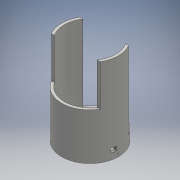
# Autodesk Inventor part: outsideCover
Saved by Autodesk Inventor 2016 (Build 200138000, 138)
## iProperties
Created: 2016-10-27
Part Number: outsideCover
Material: 一般
Document SubType Name: Modeling
Designer: Daisuke
Density: 1 g/cm^3
Appearance: 既定
Author: Daisuke
Autodesk Inventor part; units mm, degrees
ref_plane "XY Plane" through (0, 0, 0) normal (0, 0, 1) x (1, 0, 0)
sketch "スケッチ1" plane through (0, 0, 0) normal (0, 0, 1) x (1, 0, 0)
  circle A0 centre (0, 0) radius 50
  circle A1 centre (0, 0) radius 55
  line L0 (0, 0) -> (47.6314, 27.5) construction
  line L1 (0, 0) -> (55, 0) construction
  line L2 (0, 0) -> (-47.6314, 27.5) construction
  line L3 (0, 0) -> (55, 0) construction
  dimension "d0" = 100
  dimension "d1" = 110
  dimension "d2" = 30
  dimension "d3" = 150
  constraints: 8 end point, 2 centre point, 2 coincident, 2 equal length, 2 horizontal, 2 point on circle
  measures "d0" diameter of A0
  measures "d1" diameter of A1
  measures "d2" angle of L1 L0
  measures "d3" angle of L3 L2
extrude "押し出し1" add sketch "スケッチ1" along normal blind 20
sketch "スケッチ2" plane through (0, 0, 20) normal (0, 0, 1) x (1, 0, 0)
  line L0 (0, 0) -> (47.6314, 27.5) construction
  circle A0 centre (0, 0) radius 55 construction
  line L1 (0, 0) -> (55, 0) construction
  line L2 (0, 0) -> (-47.6314, 27.5) construction
  line L3 (0, 0) -> (55, 0) construction
  line L4 (-47.6314, 27.5) -> (-41.7582, 27.5)
  line L5 (41.7582, 27.5) -> (47.6314, 27.5)
  line L6 (0, 0) -> (47.6314, -27.5) construction
  line L7 (0, 0) -> (55, 0) construction
  line L8 (0, 0) -> (-47.6314, -27.5) construction
  line L9 (0, 0) -> (55, 0) construction
  arc A1 (-47.6314, 27.5) -> (-47.6314, -27.5) centre (0, 0) ccw
  arc A2 (47.6314, -27.5) -> (47.6314, 27.5) centre (0, 0) ccw
  arc A3 (-41.7582, 27.5) -> (-41.7582, -27.5) centre (0, 0) ccw
  arc A4 (41.7582, -27.5) -> (41.7582, 27.5) centre (0, 0) ccw
  line L10 (-47.6314, -27.5) -> (-41.7582, -27.5)
  line L11 (41.7582, -27.5) -> (47.6314, -27.5)
  dimension "d6" = 30
  dimension "d7" = 150
  dimension "d43" = 30
  dimension "d44" = 150
  constraints: 24 end point, 12 point on circle, 4 centre point, 4 equal length, 4 horizontal, 2 coincident
  measures "d6" angle of L1 L0
  measures "d7" angle of L3 L2
  measures "d43" angle of L6 L7
  measures "d44" angle of L8 L9
ref_plane "作業平面1" through (55, 0, 0) normal (1, 0, 0) x (0, 1, 0)
ref_plane "作業平面2" through (-55, 0, 0) normal (1, 0, 0) x (0, 1, 0)
ref_plane "作業平面3" through (0, 55, 0) normal (0, 1, 0) x (-1, 0, 0)
ref_plane "作業平面4" through (0, -55, 0) normal (0, 1, 0) x (-1, 0, 0)
sketch "スケッチ3" plane through (55, 0, 0) normal (1, 0, 0) x (0, 1, 0)
  line L0 (0, 0) -> (0, 4) construction
  circle A0 centre (0, 4) radius 1.5
  dimension "d14" = 4
  dimension "d15" = 3
  constraints: 2 end point, 1 centre point, 1 coincident, 1 vertical
  measures "d14" distance of L0.start L0.end
  measures "d15" diameter of A0
extrude "押し出し3" cut sketch "スケッチ3" against normal blind 6
sketch "スケッチ4" plane through (0, 55, 0) normal (0, 1, 0) x (-1, 0, 0)
  line L0 (0, 0) -> (0, 4) construction
  circle A0 centre (0, 4) radius 1.5
  dimension "d18" = 4
  dimension "d19" = 3
  constraints: 2 end point, 1 centre point, 1 coincident, 1 vertical
  measures "d18" distance of L0.start L0.end
  measures "d19" diameter of A0
extrude "押し出し4" cut sketch "スケッチ4" against normal blind 6
sketch "スケッチ5" plane through (-55, 0, 0) normal (1, 0, 0) x (0, 1, 0)
  line L0 (0, 0) -> (0, 4) construction
  circle A0 centre (0, 4) radius 1.5
  dimension "d22" = 4
  dimension "d23" = 3
  constraints: 2 end point, 1 centre point, 1 coincident, 1 vertical
  measures "d22" distance of L0.start L0.end
  measures "d23" diameter of A0
extrude "押し出し5" cut sketch "スケッチ5" along normal blind 6
sketch "スケッチ6" plane through (0, -55, 0) normal (0, 1, 0) x (-1, 0, 0)
  line L0 (0, 0) -> (0, 4) construction
  circle A0 centre (0, 4) radius 1.5
  dimension "d26" = 4
  dimension "d27" = 3
  constraints: 2 end point, 1 centre point, 1 coincident, 1 vertical
  measures "d26" distance of L0.start L0.end
  measures "d27" diameter of A0
extrude "押し出し6" cut sketch "スケッチ6" along normal blind 6
ref_plane "作業平面5" through (55, 0, 0) normal (1, 0, 0) x (0, 1, 0)
extrude "押し出し9" add sketch "スケッチ2" along normal blind 150.5
sketch "スケッチ8" plane through (0, 0, 20) normal (0, 0, 1) x (1, 0, 0)
  line L0 (-47.6314, -27.5) -> (-41.7582, -27.5) projected
  arc A0 (-47.6314, -27.5) -> (47.6314, -27.5) centre (0, 0) ccw
  arc A1 (-41.7582, -27.5) -> (41.7582, -27.5) centre (0, 0) ccw projected
  arc A2 (41.7582, -27.5) -> (41.7582, -27.5) centre (0, 0) ccw
  line L1 (-47.6314, -27.5) -> (-41.7582, -27.5)
  line L2 (41.7582, -27.5) -> (47.6314, -27.5)
  constraints: 4 end point, 4 point on circle, 2 centre point, 2 coincident, 1 collinear, 1 horizontal
extrude "押し出し10" add sketch "スケッチ8" along normal blind 70.5 contours L0 A1 L2 A0
sketch "スケッチ9" plane through (55, 0, 0) normal (1, 0, 0) x (0, 1, 0)
  line L0 (0, 0) -> (0, 12) construction
  line L1 (0, 12) -> (-3.5, 12) construction
  line L2 (-3.5, 12) -> (-13.5, 12)
  line L3 (-13.5, 12) -> (-13.5, 20)
  line L4 (-13.5, 20) -> (-3.5, 20)
  line L5 (-3.5, 20) -> (-3.5, 12)
  dimension "d49" = 12
  dimension "d50" = 3.5
  dimension "d51" = 10
  dimension "d52" = 8
  constraints: 12 end point, 2 horizontal, 2 parallel, 1 perpendicular, 1 vertical
  measures "d49" distance of L0.start L0.end
  measures "d50" distance of L0.end L1.end
  measures "d51" distance of L3.end L4.end
  measures "d52" distance of L2.end L3.end
extrude "押し出し11" cut sketch "スケッチ9" against normal blind 10
